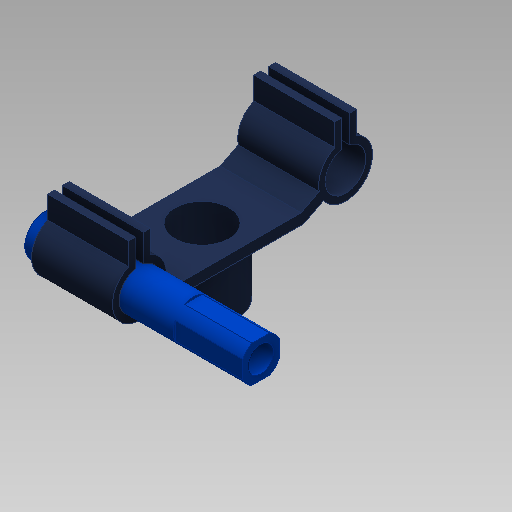
# Autodesk Inventor part: B8-A4
Saved by Autodesk Inventor 2018.1 (Build 221171000, 171)
## iProperties
Created: 2018-06-23
Part Number: B8-A4
Material: Všeobecné
Document SubType Name: Modeling
Designer: PS
Density: 1 g/cm^3
Appearance: Výchozí
Author: PS
Autodesk Inventor part; units mm, degrees
ref_plane "YZ Plane" through (0, 0, 0) normal (1, 0, 0) x (0, 1, 0)
ref_plane "XZ Plane" through (0, 0, 0) normal (0, 1, 0) x (-1, 0, 0)
ref_plane "XY Plane" through (0, 0, 0) normal (0, 0, 1) x (1, 0, 0)
sketch "Náčrt1" plane through (0, 0, 0) normal (0, 0, 1) x (1, 0, 0)
  point P0 (0, 0)
sketch "Náčrt2" plane through (0, 0, 0) normal (0, 0, 1) x (1, 0, 0)
  circle A0 centre (0, 0) radius 20
  circle A1 centre (0, 0) radius 26
  dimension "d0" = 40
  dimension "d1" = 6
  constraints: 2 centre point, 1 coincident
  measures "d0" diameter of A0
  measures "d1" radial gap between concentric circles of A0 A1
extrude "Vysunutí1" add sketch "Náčrt2" along normal blind 40
sketch "Náčrt3" plane through (0, 0, 0) normal (1, 0, 0) x (0, 1, 0)
  line L0 (26, 40) -> (-26, 40) projected
  line L1 (0, 40) -> (-45.414, 40)
  line L2 (-45.414, 40) -> (-62.0898, 48.5204)
  line L3 (-58.9679, 55.909) -> (-43.4886, 48)
  line L4 (-43.4886, 48) -> (0, 48)
  arc A0 (-79.4326, 78.7082) -> (-73.4326, 78.7082) centre (-76.4326, 58.9345) ccw
  line L5 (-58.9679, 55.909) -> (-62.0898, 48.5204)
  line L6 (-60.5289, 52.2147) -> (-76.4326, 58.9345) construction
  line L7 (-76.4326, 58.9345) -> (-76.4326, 91.1664) construction
  line L8 (-79.4326, 93.9345) -> (-84.4326, 93.9345)
  line L9 (-84.4326, 93.9345) -> (-84.4326, 73.6314)
  line L10 (-84.4326, 73.6314) -> (-79.4326, 73.6314)
  line L11 (-79.4326, 73.6314) -> (-79.4326, 93.9345)
  line L12 (-73.4326, 73.6314) -> (-68.4326, 73.6314)
  line L13 (-68.4326, 73.6314) -> (-68.4326, 93.9345)
  line L14 (-68.4326, 93.9345) -> (-73.4326, 93.9345)
  line L15 (-73.4326, 93.9345) -> (-73.4326, 73.6314)
  arc A1 (-79.4326, 73.6314) -> (-73.4326, 73.6314) centre (-76.4326, 58.9345) ccw
  line L16 (0, 48) -> (0, 40)
  point P0 (0, 0)
  dimension "d4" = 8
  dimension "d5" = 40
  dimension "d7" = 5
  dimension "d8" = 6
  dimension "d9" = 3
  dimension "d10" = 15
  constraints: 32 end point, 4 parallel, 4 perpendicular, 4 point on circle, 3 collinear, 3 horizontal, 2 centre point, 2 coincident, 2 midpoint, 2 point on line, 1 vertical, 1 other
  measures "d4" distance between parallel lines of L2 L3
  measures "d5" diameter of A0
  measures "d7" distance of L8.start L8.end
  measures "d8" distance between parallel lines of L15 L11
  measures "d9" distance between parallel lines of L11 L7
  measures "d10" distance edge to line of A0 L8
extrude "Vysunutí2" add sketch "Náčrt3" along normal mid plane 60
mirror "Zrcadlit1" about plane through (0, 0, 0) normal (0, 1, 0) of "Vysunutí2"
sketch "Náčrt4" plane through (-30, -43.4886, 48) normal (0, 0, 1) x (1, 0, 0)
  circle A0 centre (30, 43.4886) radius 20 projected
extrude "Vysunutí3" cut sketch "Náčrt4" against normal blind 40
sketch "Náčrt5" plane through (30, 0, 0) normal (1, 0, 0) x (0, 0, -1)
  arc A0 (-73.6314, -79.4326) -> (-73.6314, -73.4326) centre (-58.9345, -76.4326) ccw projected
  circle A1 centre (-58.9345, -76.4326) radius 15
  circle A2 centre (-58.9345, -76.4326) radius 9.5
  point P0 (0, 0)
  dimension "d15" = 19
  constraints: 2 coincident, 1 centre point, 3 other
  measures "d15" diameter of A2
extrude "Vysunutí4" add sketch "Náčrt5" along normal blind 90 and the other way blind 70 separate body
sketch "Náčrt6" plane through (120, -76.4326, 58.9345) normal (1, 0, 0) x (0, 0, -1)
  line L0 (13.5, -13.5) -> (-13.5, -13.5)
  line L1 (-13.5, -13.5) -> (-13.5, 13.5)
  line L2 (-13.5, 13.5) -> (13.5, 13.5)
  line L3 (13.5, 13.5) -> (13.5, -13.5)
  line L4 (13.5, -13.5) -> (-13.5, 13.5) construction
  line L5 (-13.5, -13.5) -> (13.5, 13.5) construction
  circle A0 centre (0, 0) radius 9.5 projected
  line L6 (-20.2709, 20.2709) -> (-20.2709, -20.2709)
  line L7 (-20.2709, -20.2709) -> (20.2709, -20.2709)
  line L8 (20.2709, -20.2709) -> (20.2709, 20.2709)
  line L9 (20.2709, 20.2709) -> (-20.2709, 20.2709)
  point P0 (58.9345, 76.4326)
  dimension "d20" = 27
  constraints: 20 end point, 4 parallel, 3 perpendicular, 2 midpoint, 1 coincident, 1 horizontal, 3 other
  measures "d20" distance of L2.end L0.start
extrude "Vysunutí5" cut sketch "Náčrt6" against normal blind 50 contours L9 L8 L7 L6 bodies 2
equation "\"d9\" = 0.5 * d8"
